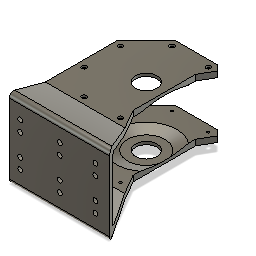
StandSupport (Autodesk Fusion 360 design; units mm, degrees)
Autodesk Fusion 360 part; units mm, degrees
sketch "Sketch1" plane through (0, 0, 0) normal (1, 0, 0) x (0, 0, -1)
  line L0 (70, -35) -> (-71.0532, -35)
  line L1 (-71.0532, -35) -> (-110, -45.4358)
  line L2 (-110, -45.4358) -> (-110, 45.4358)
  line L3 (-110, 45.4358) -> (-71.0532, 35)
  line L4 (-71.0532, 35) -> (70, 35)
  line L5 (70, 35) -> (70, 43)
  line L6 (70, 43) -> (-70, 43)
  line L7 (-70, 43) -> (-112.4471, 54.3737)
  line L8 (-120, 48.5781) -> (-120, -48.5781)
  line L9 (-112.4471, -54.3737) -> (-70, -43)
  line L10 (-70, -43) -> (70, -43)
  line L11 (70, -43) -> (70, -35)
  line L12 (-70, 35) -> (70, 35)
  line L13 (-70, -35) -> (70, -35)
  line L14 (0, 0) -> (-38.2149, 0) construction
  arc A0 (-112.4471, 54.3737) -> (-120, 48.5781) centre (-114, 48.5781) ccw
  arc A1 (-120, -48.5781) -> (-112.4471, -54.3737) centre (-114, -48.5781) ccw
  dimension "d50" = 8
  dimension "d51" = 110
  dimension "d52" = 10
  dimension "d53" = 8
  dimension "d54" = 8
  dimension "d55" = 75
  dimension "d56" = 6
  constraint horizontal L0
  constraint vertical L2
  constraint horizontal L4
  constraint perpendicular L4 L5
  constraint perpendicular L5 L6
  constraint perpendicular L4 L8
  constraint perpendicular L8 L10
  constraint coincident L4.end L12
  constraint coincident L5 L4.end
  constraint coincident L0.start L13
  constraint coincident L11 L0.start
  constraint perpendicular L0 L11
  constraint equal L5 L11
  constraint parallel L1 L9
  constraint parallel L3 L7
  constraint coincident L14.start origin
  constraint horizontal L14
  constraint symmetric L1 L3 L14
  constraint vertical L6.end L12.start
  constraint tangent L7 A0
  constraint tangent L8 A0
  constraint tangent L8 A1
  constraint tangent L9 A1
  constraint equal A0 A1
  measures "d50" distance of L0.start L10.end L5.end
  measures "d51" distance of L14.start L2
  measures "d52" distance of L2 L8
  measures "d53" distance of L1 L9
  measures "d54" distance of L3 L7
  measures "d55" angle of L2 L3
  measures "d56" radius of A0
extrude "Extrude1" add sketch "Sketch1" along normal blind -70 and the other way blind -70
sketch "Sketch2" plane through (0, -43, 0) normal (0, -1, 0) x (1, 0, 0)
  line L0 (70, 70) -> (-70, 70)
  line L1 (-70, 70) -> (-70, -70)
  line L2 (-70, -70) -> (70, -70)
  line L3 (70, -70) -> (70, 70)
  line L4 (-70, -28.9949) -> (-28.9949, -70)
  line L5 (28.9949, -70) -> (70, -28.9949)
  line L6 (0, 0) -> (0, -43.9465) construction
  line L7 (-28.9949, -70) -> (28.9949, -70)
  constraint coincident L1 L4.start
  constraint coincident L2 L4.end
  constraint coincident L2 L5.start
  constraint coincident L3 L5.end
  constraint coincident L6.start origin
  constraint parallel L1 L6
  constraint symmetric L4 L5 L6
  constraint perpendicular L4 L5
  constraint equal L5 L7
extrude "Extrude2" cut sketch "Sketch2" against normal up to surface (86 mm away) contours L2 L3 L5 | L1 L2 L4
sketch "Sketch3" plane through (0, -43, 0) normal (0, -1, 0) x (1, 0, 0)
  line L0 (-70, -28.9949) -> (-28.9949, -70)
  line L1 (-28.9949, -70) -> (28.9949, -70)
  line L2 (28.9949, -70) -> (70, -28.9949)
  line L3 (70, -28.9949) -> (70, 70)
  line L4 (70, 70) -> (-70, 70)
  line L5 (-70, 70) -> (-70, -28.9949)
  circle A0 centre (0, 0) radius 15
  dimension "d63" = 30
  constraint coincident A0.centre origin
  measures "d63" diameter of A0
extrude "Extrude3" cut sketch "Sketch3" against normal up to surface (86 mm away) contours A0
sketch "Sketch4" plane through (0, -43, 0) normal (0, -1, 0) x (1, 0, 0)
  circle A0 centre (0, 0) radius 15
  line L0 (-70, -28.9949) -> (-28.9949, -70)
  line L1 (-28.9949, -70) -> (28.9949, -70)
  line L2 (28.9949, -70) -> (70, -28.9949)
  line L3 (70, -28.9949) -> (70, 70)
  line L4 (70, 70) -> (-70, 70)
  line L5 (-70, 70) -> (-70, -28.9949)
  line L6 (0, 0) -> (36.2347, -62.7603)
  line L7 (0, 0) -> (117.4674, 0) construction
  line L8 (0, 0) -> (70, 121.2436)
  line L9 (25, 43.3013) -> (25, -43.3013)
  line L10 (70, 70) -> (70, 121.2436)
  dimension "d67" = 120
  dimension "d68" = 25
  constraint coincident A0.centre L6.start
  constraint coincident L2 L6.end
  constraint perpendicular L3 L7
  constraint coincident L3 L8.end
  constraint coincident L8 L9.start
  constraint coincident L6 L9.end
  constraint vertical L9
  constraint coincident L3.end L4.start
  measures "d67" angle of L6 L8
  measures "d68" distance of A0.centre L9
extrude "Extrude4" cut sketch "Sketch4" along normal up to surface (-106 mm away) and the other way blind -20 contours L2 L3 L4 L6 L8 L9 | L4 L8 L10
sketch "Sketch5" plane through (0, -35, 0) normal (0, 1, 0) x (-1, 0, 0)
  line L0 (-41.0226, 71.0532) -> (-25, 43.3013)
  line L1 (-25, 43.3013) -> (-25, -43.3013)
  line L2 (-25, -43.3013) -> (-36.2347, -62.7603)
  line L3 (-36.2347, -62.7603) -> (-28.9949, -70)
  line L4 (-28.9949, -70) -> (28.9949, -70)
  line L5 (28.9949, -70) -> (70, -28.9949)
  line L6 (70, -28.9949) -> (70, 71.0532)
  line L7 (70, 71.0532) -> (-41.0226, 71.0532)
  circle A0 centre (0, 0) radius 15
  circle A1 centre (0, 0) radius 26
  dimension "d73" = 52
  constraint coincident A0.centre A1.centre
  measures "d73" diameter of A1
extrude "Extrude5" cut sketch "Sketch5" along normal up to surface (74 mm away) and the other way blind 4 contours L1 A1 picked at (-21.6667, 0)
chamfer "Chamfer1" distance 16 distance2 4 2 edges at (-26, -35, 0) (-26, 35, 0) measured on face at (-55.124, -35, 15.9129) measured on face at (-55.124, 35, 15.9129)
sketch "Sketch6" plane through (0, 43, 0) normal (0, 1, 0) x (-1, 0, 0)
  line L0 (-40.4145, 70) -> (-25, 43.3013)
  line L1 (-25, 43.3013) -> (-25, -43.3013)
  line L2 (-25, -43.3013) -> (-36.2347, -62.7603)
  line L3 (-36.2347, -62.7603) -> (-28.9949, -70)
  line L4 (-28.9949, -70) -> (28.9949, -70)
  line L5 (28.9949, -70) -> (70, -28.9949)
  line L6 (70, -28.9949) -> (70, 70)
  line L7 (70, 70) -> (-40.4145, 70)
  circle A0 centre (0, 0) radius 15
  circle A1 centre (-25.2571, 60.976) radius 1.7
  circle A2 centre (25.2571, -60.976) radius 1.7
  circle A3 centre (60.976, -25.2571) radius 1.7
  circle A4 centre (-60.976, 25.2571) radius 1.7
  circle A5 centre (25.2571, 60.976) radius 1.7
  circle A6 centre (-25.2571, -60.976) radius 1.7
  circle A7 centre (60.976, 25.2571) radius 1.7
  circle A8 centre (-60.976, -25.2571) radius 1.7
  circle A9 centre (0, 0) radius 42
  circle A10 centre (0, 0) radius 70
extrude "Extrude6" cut sketch "Sketch6" against normal up to surface (86 mm away) contours A1 | A2 | A3 | A5 | A6 | A7
sketch "Sketch7" plane through (0, 0, 120) normal (0, 0, 1) x (1, 0, 0)
  line L0 (69.282, -48.5781) -> (69.282, 48.5781)
  line L1 (69.282, 48.5781) -> (-70, 48.5781)
  line L2 (-70, 48.5781) -> (-70, -48.5781)
  line L3 (-70, -48.5781) -> (69.282, -48.5781)
  line L4 (-70, 0) -> (44.2317, 0) construction
  circle A0 centre (-55, 15) radius 3.25
  circle A1 centre (49.282, 15) radius 3.25
  circle A2 centre (-55, 30) radius 3.25
  circle A3 centre (49.282, 30) radius 3.25
  circle A4 centre (0, 30) radius 3.25
  circle A5 centre (0, 15) radius 3.25
  circle A6 centre (-55, -30) radius 3.25
  circle A7 centre (-55, -15) radius 3.25
  circle A8 centre (0, -30) radius 3.25
  circle A9 centre (0, -15) radius 3.25
  circle A10 centre (49.282, -30) radius 3.25
  circle A11 centre (49.282, -15) radius 3.25
  dimension "d82" = 15
  dimension "d83" = 6.5
  dimension "d84" = 30
  dimension "d85" = 15
  dimension "d86" = 20
  constraint midpoint L2 L4.start
  constraint perpendicular L2 L4
  constraint horizontal A0.centre A1.centre
  constraint equal A0 A1
  constraint vertical A0.centre A2.centre
  constraint horizontal A2.centre A3.centre
  constraint vertical A1.centre A3.centre
  constraint equal A0 A2
  constraint equal A0 A3
  constraint vertical A4.centre A5.centre
  constraint horizontal A0.centre A5.centre
  constraint horizontal A2.centre A4.centre
  constraint vertical origin A5.centre
  constraint equal A0 A5
  constraint equal A0 A4
  constraint symmetric L4 A0 A7
  constraint symmetric L4 A1 A11
  constraint symmetric L4 A2 A6
  constraint symmetric L4 A3 A10
  constraint symmetric L4 A4 A8
  constraint symmetric L4 A5 A9
  measures "d82" distance of L4 A0.centre
  measures "d83" diameter of A0
  measures "d84" distance of L4 A2.centre
  measures "d85" distance of L2 A2.centre
  measures "d86" distance of L0 A3.centre
extrude "Extrude7" cut sketch "Sketch7" against normal up to surface (10 mm away) contours A0 | A1 | A2 | A3 | A4 | A5 | A6 | A7 | A8 | A9 | A10 | A11
sketch "Sketch8" plane through (0, 43, 0) normal (0, 1, 0) x (-1, 0, 0)
  circle A0 centre (60.976, 25.2571) radius 1.7
  circle A1 centre (25.2571, -60.976) radius 1.7
  circle A2 centre (25.2571, 60.976) radius 1.7
  circle A3 centre (60.976, -25.2571) radius 1.7
  circle A4 centre (-25.2571, -60.976) radius 1.7
  circle A5 centre (-25.2571, 60.976) radius 1.7
  line L0 (-40.4145, 70) -> (-25, 43.3013)
  line L1 (-25, 43.3013) -> (-25, -43.3013)
  line L2 (-25, -43.3013) -> (-36.2347, -62.7603)
  line L3 (-36.2347, -62.7603) -> (-28.9949, -70)
  line L4 (-28.9949, -70) -> (28.9949, -70)
  line L5 (28.9949, -70) -> (70, -28.9949)
  line L6 (70, -28.9949) -> (70, 70)
  line L7 (70, 70) -> (-40.4145, 70)
  circle A6 centre (0, 0) radius 15
  circle A7 centre (25.2571, -60.976) radius 3.25
  circle A8 centre (60.976, -25.2571) radius 3.25
  circle A9 centre (60.976, 25.2571) radius 3.25
  circle A10 centre (25.2571, 60.976) radius 3.25
  circle A11 centre (-25.2571, 60.976) radius 3.25
  circle A12 centre (-60.976, 25.2571) radius 3.25
  circle A13 centre (-60.976, -25.2571) radius 3.25
  circle A14 centre (-25.2571, -60.976) radius 3.25
  dimension "d89" = 6.5
  dimension "d91" = 360
  constraint concentric A1 A7
  measures "d89" diameter of A7
extrude "Extrude8" cut sketch "Sketch8" against normal blind 3 contours A7 | A8 | A9 | A10 | A11 | A14
mirror "Mirror1" about plane through (0, 0, 0) normal (0, 1, 0) of "Extrude8"
chamfer "Chamfer2" distance 4 distance2 3 2 edges at (-3.2457, 45.4358, 110) (-3.2457, -45.4358, 110) measured on face at (-19.3094, -4.53, 110) measured on face at (11.5104, -41.9572, 97.0177)
